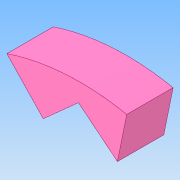
# Autodesk Inventor part: BearingHolder2
Saved by Autodesk Inventor 2017.3 (Build 213256000, 256)
## iProperties
Created: 2019-06-19
Part Number: BearingHolder2
Material: ABS Plastic
Document SubType Name: Modeling
Designer: Derek Wider
Density: 1.06 g/cm^3
Appearance: Pink
Author: Derek Wider
Autodesk Inventor part; units mm, degrees
ref_plane "YZ Plane" through (0, 0, 0) normal (1, 0, 0) x (0, 1, 0)
ref_plane "XZ Plane" through (0, 0, 0) normal (0, 1, 0) x (-1, 0, 0)
ref_plane "XY Plane" through (0, 0, 0) normal (0, 0, 1) x (1, 0, 0)
sketch "Sketch1" plane through (0, 0, 0) normal (0, 0, 1) x (1, 0, 0)
  line L0 (0, 0) -> (4.826, 4.3221)
  line L1 (4.826, 4.3221) -> (10.16, 0)
  line L2 (10.16, 0) -> (11.43, 6.2217)
  line L3 (0, 0) -> (-4.975, 5.229)
  arc A0 (11.43, 6.2217) -> (-4.975, 5.229) centre (5.08, -24.8868) ccw
  circle A1 centre (5.08, -24.8868) radius 25.4 construction
  circle A2 centre (5.08, -24.8868) radius 21.59 construction
  circle A3 centre (5.08, -49.6518) radius 1.5875
  line L4 (5.08, -49.6518) -> (5.08, -46.4768) construction
  line L5 (0, 0) -> (0, -3.2502)
  circle A4 centre (5.08, -24.8868) radius 22.225
  circle A5 centre (5.08, -49.6518) radius 3.81
  dimension "d40" = 43.18
  dimension "d0" = 31.75
  dimension "d2" = 50.8
  dimension "d3" = 29.21
  dimension "d4" = 30
  dimension "d5" = 10.16
  dimension "d6" = 5.334
  dimension "d43" = 3.175
  dimension "d44" = 3.175
  dimension "d53" = 44.45
  dimension "d54" = 7.62
  constraints: 12 end point, 5 centre point, 4 point on circle, 3 coincident, 2 vertical, 2 vertical alignment, 1 horizontal alignment, 1 line through centre, 2 other
  measures "d0" radius of A0
  measures "d2" diameter of A1
  measures "d3" distance of A1.centre L0.end
  measures "d5" distance of L1.end L0.start
  measures "d6" horizontal distance of L1.end L0.end
  measures "d43" diameter of A3
  measures "d44" distance of L4.start L4.end
  measures "d53" diameter of A4
  measures "d54" diameter of A5
extrude "Extrusion1" add sketch "Sketch1" along normal blind 6.35 contours L3 A0 L2 L1 L0
body "Solid1"
